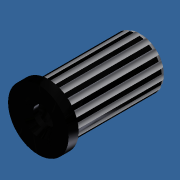
# Autodesk Inventor part: shaft-gear
Saved by Autodesk Inventor 2015 (Build 190159000, 159)
## iProperties
Created: 2019-04-15
Part Number: shaft-gear
Material: Generic
Document SubType Name: Modeling
Designer: gabriel
Density: 1 g/cm^3
Appearance: Default
Author: gabriel
Autodesk Inventor part; units mm, degrees
ref_plane "YZ Plane" through (0, 0, 0) normal (1, 0, 0) x (0, 1, 0)
ref_plane "XZ Plane" through (0, 0, 0) normal (0, 1, 0) x (-1, 0, 0)
ref_plane "XY Plane" through (0, 0, 0) normal (0, 0, 1) x (1, 0, 0)
sketch "Sketch20" plane through (0, 0, 0) normal (0, 0, 1) x (1, 0, 0)
  line L0 (2.8871, 0) -> (1.4436, -2.5003)
  line L1 (1.4436, -2.5003) -> (-1.4436, -2.5003)
  line L2 (-1.4436, -2.5003) -> (-2.8871, 0)
  line L3 (-2.8871, 0) -> (-1.4436, 2.5003)
  line L4 (-1.4436, 2.5003) -> (1.4436, 2.5003)
  line L5 (1.4436, 2.5003) -> (2.8871, 0)
  circle A0 centre (0, 0) radius 3.9688
  dimension "d79" = 5.0006
  dimension "d89" = 7.9375
  constraints: 12 end point, 3 coincident, 1 centre point, 1 horizontal, 13 other
  measures "d79" distance between parallel lines of L1 L4
  measures "d89" diameter of A0
extrude "Extrusion19" add sketch "Sketch20" along normal blind 14.6844
sketch "Sketch25" plane through (0, 0, 14.6844) normal (0, 0, 1) x (1, 0, 0)
  circle A0 centre (0, 0) radius 3.9687 projected
  circle A1 centre (3.9687, 0) radius 0.4536
  circle A2 centre (3.6666, 1.5188) radius 0.4536
  circle A3 centre (2.8063, 2.8063) radius 0.4536
  circle A4 centre (1.5188, 3.6666) radius 0.4536
  circle A5 centre (0, 3.9687) radius 0.4536
  circle A6 centre (-1.5188, 3.6666) radius 0.4536
  circle A7 centre (-2.8063, 2.8063) radius 0.4536
  circle A8 centre (-3.6666, 1.5188) radius 0.4536
  circle A9 centre (-3.9687, 0) radius 0.4536
  circle A10 centre (-3.6666, -1.5188) radius 0.4536
  circle A11 centre (-2.8063, -2.8063) radius 0.4536
  circle A12 centre (-1.5188, -3.6666) radius 0.4536
  circle A13 centre (0, -3.9687) radius 0.4536
  circle A14 centre (1.5188, -3.6666) radius 0.4536
  circle A15 centre (2.8063, -2.8063) radius 0.4536
  circle A16 centre (3.6666, -1.5188) radius 0.4536
  dimension "d155" = 0.9071
  dimension "d158" = 360
  constraints: 16 centre point, 2 horizontal alignment, 34 other
  measures "d155" diameter of A1
sketch "Sketch36" plane through (0, 0, 14.6844) normal (0, 0, 1) x (1, 0, 0)
  circle A0 centre (0, 0) radius 4.7625
  dimension "d144" = 9.525
  constraints: 1 centre point, 1 coincident
  measures "d144" diameter of A0
extrude "Extrusion34" add sketch "Sketch36" along normal blind 1.5875
sketch "Sketch37" plane through (0, 0, 16.2719) normal (0, 0, 1) x (1, 0, 0)
  circle A0 centre (0, 0) radius 1.5875
  dimension "d147" = 3.175
  constraints: 1 centre point, 1 coincident
  measures "d147" diameter of A0
extrude "Extrusion35" cut sketch "Sketch37" against normal through all
chamfer "Chamfer5" distance 0.7937 angle 45 1 edges at (-1.5875, 0, 16.2719)
fillet "Fillet2" radius 0.7937 1 edges at (-3.9688, 0, 0)
extrude "Extrusion39" cut sketch "Sketch25" against normal up to next contours A0 A1 | A0 A1 | A2 A0 | A0 A2 | A16 A0 | A0 A16 | A3 A0 | A0 A3 | A15 A0 | A0 A15 | A4 A0 | A0 A4 | A14 A0 | A0 A14 | A5 A0 | A0 A5 | A13 A0 | A0 A13 | A6 A0 | A0 A6 | A12 A0 | A0 A12 | A7 A0 | A0 A7 | A11 A0 | A0 A11 | A8 A0 | A0 A8 | A10 A0 | A0 A10 | A9 A0 | A0 A9
equation "\"d27\" = 0.5 * d26"
equation "\"d26\" = 3.175"
body "Solid5"
